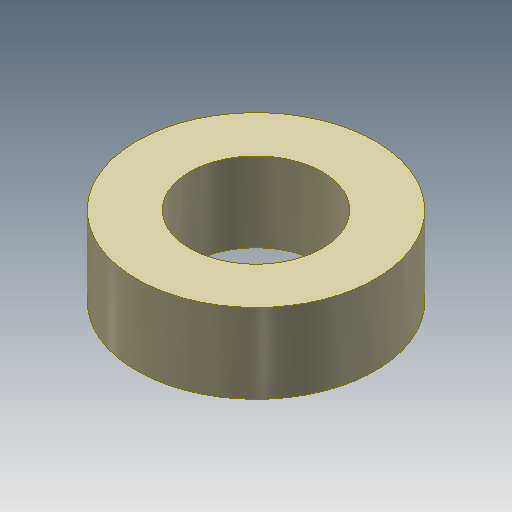
# Autodesk Inventor part: Nema 17 Plastic Spacer 2
Saved by Autodesk Inventor 2020.2 (Build 242310000, 310)
## iProperties
Created: 2020-01-17
Part Number: Nema 17 Plastic Spacer 2
Material: Nylon 6/6
Document SubType Name: Modeling
Designer: james
Density: 1.13 g/cm^3
Appearance: Nylon 6
Mass: 0.1491 g
Surface Area: 2.19911 cm^2
Volume: 0.131947 cm^3
Author: james
Autodesk Inventor part; units mm, degrees
ref_plane "YZ Plane" through (0, 0, 0) normal (1, 0, 0) x (0, 1, 0)
ref_plane "XZ Plane" through (0, 0, 0) normal (0, 1, 0) x (-1, 0, 0)
ref_plane "XY Plane" through (0, 0, 0) normal (0, 0, 1) x (1, 0, 0)
sketch "Sketch11" plane through (0, 0, 0) normal (0, 1, 0) x (-1, 0, 0)
  circle A0 centre (0, 0) radius 2.5
  circle A1 centre (0, 0) radius 4.5
  dimension "d82" = 5
  dimension "d83" = 9
  constraints: 2 centre point, 2 coincident
  measures "d82" diameter of A0
  measures "d83" diameter of A1
extrude "Extrusion7" add sketch "Sketch11" along normal mid plane 3
body "Solid6"
